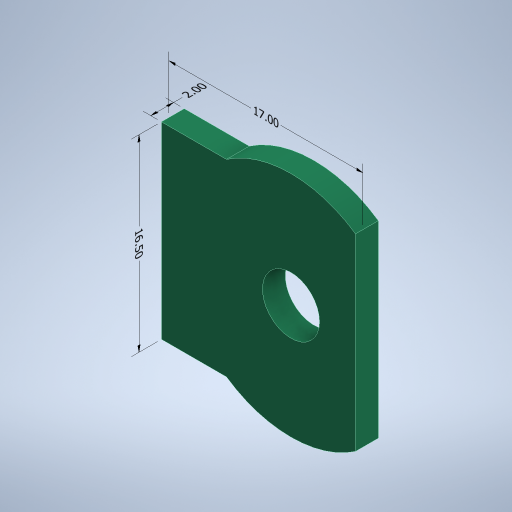
# Autodesk Inventor part: encoder
Saved by Autodesk Inventor 2024.1 (Build 281209000, 209)
## iProperties
Created: 2024-07-01
Part Number: encoder
Material: 一般
Document SubType Name: Modeling
Designer: hibik
Density: 1 g/cm^3
Appearance: 既定
Author: hibik
Autodesk Inventor part; units mm, degrees
ref_plane "YZ Plane" through (0, 0, 0) normal (1, 0, 0) x (0, 1, 0)
ref_plane "XZ Plane" through (0, 0, 0) normal (0, 1, 0) x (-1, 0, 0)
ref_plane "XY Plane" through (0, 0, 0) normal (0, 0, 1) x (1, 0, 0)
sketch "スケッチ1" plane through (0, 0, 0) normal (0, 0, 1) x (1, 0, 0)
  circle A0 centre (0, 0) radius 10
  line L0 (-11.3487, 8.25) -> (5.6513, 8.25)
  line L1 (5.6513, 8.25) -> (5.6513, -8.25)
  line L2 (5.6513, -8.25) -> (-11.3487, -8.25)
  line L3 (-11.3487, -8.25) -> (-11.3487, 8.25)
  point P0 (5.6513, 0)
  point P1 (-5.6513, 8.25)
  point P2 (-5.6513, -8.25)
  dimension "d0" = 20
  dimension "d1" = 16.5
  dimension "d2" = 17
  constraints: 8 end point, 2 parallel, 1 coincident, 1 horizontal, 1 horizontal alignment, 1 midpoint, 1 perpendicular, 3 other
  measures "d1" distance of L0.end L1.end
  measures "d2" distance of L0.start L0.end
extrude "押し出し1" add sketch "スケッチ1" along normal blind 2 contours L0 A0 | L1 L2 A0 L0 | A0 L2 | A0 L2 L3 L0
sketch "スケッチ2" plane through (0, 0, 2) normal (0, 0, 1) x (1, 0, 0)
  circle A0 centre (0, 0) radius 2.5
  dimension "d5" = 5
  constraints: 1 centre point, 1 coincident
  measures "d5" diameter of A0
extrude "押し出し2" cut sketch "スケッチ2" against normal blind 2
